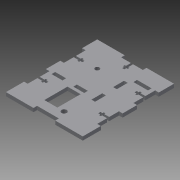
# Autodesk Inventor part: side-right
Saved by Autodesk Inventor 2014 (Build 180170000, 170)
## iProperties
Created: 2014-03-01
Part Number: side-right
Material: 常规
Document SubType Name: Modeling
Designer: Keshuai
Density: 1 g/cm^3
Appearance: 默认
Author: Keshuai
Autodesk Inventor part; units mm, degrees
sketch "slot" plane through (0, 0, 0) normal (0, 0, 1) x (1, 0, 0)
  line L0 (-16.5, 21) -> (-13.5, 21)
  line L1 (-13.5, 9) -> (-16.5, 9)
  line L2 (-11.75, 14.2) -> (-11.75, 11.8)
  line L3 (-18.25, 11.8) -> (-18.25, 14.2)
  line L4 (-18.25, 14.2) -> (-11.75, 11.8) construction
  line L5 (-11.75, 14.2) -> (-18.25, 11.8) construction
  line L6 (-18.25, 14.2) -> (-16.5, 14.2)
  line L7 (-13.5, 14.2) -> (-11.75, 14.2)
  line L8 (-16.5, 9) -> (-16.5, 11.8)
  line L9 (-16.5, 14.2) -> (-16.5, 21)
  line L10 (-13.5, 21) -> (-13.5, 14.2)
  line L11 (-13.5, 11.8) -> (-13.5, 9)
  line L12 (-11.75, 11.8) -> (-13.5, 11.8)
  line L13 (-16.5, 11.8) -> (-18.25, 11.8)
  point P0 (-15, 21)
  point P1 (-15, 13)
  dimension "d33" = 3
  dimension "d34" = 12
  dimension "d35" = 6.5
  dimension "d36" = 2.4
  dimension "d37" = 8
  measures "d33" distance of L11.end L8.start
  measures "d34" distance of L10.start L11.end
  measures "d35" distance of L4.end L5.end
  measures "d36" distance of L5.start L4.end
  measures "d37" distance from line of L0 point (-15, 13)
sketch "草图1" plane through (0, 0, 0) normal (0, 0, 1) x (1, 0, 0)
  line L0 (8, 0) -> (28, 0) projected
  line L1 (28, 0) -> (28, 5) projected
  line L2 (8, 5) -> (28, 5) projected
  line L3 (8, 0) -> (8, 5) projected
  line L4 (33, 0) -> (33, 5) projected
  line L5 (33, 21) -> (-63, 21)
  line L6 (-63, 21) -> (-63, -95)
  line L7 (-63, -95) -> (33, -95)
  line L8 (33, -95) -> (33, 21)
  circle A0 centre (-33, -9) radius 25 construction
  line L9 (0, 0) -> (0, 5) projected
  line L10 (46.5391, -42) -> (-87.8094, -42) construction
  line L11 (-43, -42) -> (-58, -42)
  line L12 (-58, -42) -> (-58, -47)
  line L13 (-58, -47) -> (-43, -47)
  line L14 (-43, -47) -> (-43, -42)
  line L15 (-13, -42) -> (-28, -42)
  line L16 (-28, -42) -> (-28, -47)
  line L17 (-28, -47) -> (-13, -47)
  line L18 (-13, -47) -> (-13, -42)
  line L19 (-9, -106.2504) -> (-9, 32.3829) construction
  line L20 (0, -5) -> (5, -5)
  line L21 (5, -5) -> (5, -20)
  line L22 (5, -20) -> (0, -20)
  line L23 (0, -20) -> (0, -5)
  line L24 (0, -35) -> (5, -35)
  line L25 (5, -35) -> (5, -50)
  line L26 (5, -50) -> (0, -50)
  line L27 (0, -50) -> (0, -35)
  circle A1 centre (-33, -9) radius 3
  dimension "d0" = 16
  dimension "d3" = 50
  dimension "d4" = 30
  dimension "d5" = 33
  dimension "d6" = 30
  dimension "d7" = 33
  dimension "d8" = 53
  dimension "d9" = 15
  dimension "d10" = 5
  dimension "d11" = 15
  dimension "d12" = 5
  dimension "d13" = 5
  dimension "d14" = 15
  dimension "d15" = 54
  dimension "d16" = 5
  dimension "d17" = 15
  dimension "d18" = 5
  dimension "d19" = 15
  dimension "d20" = 5
  dimension "d21" = 15
  dimension "d22" = 6
  constraints: 44 end point, 11 parallel, 6 perpendicular, 5 horizontal, 2 centre point, 2 point on line, 1 coincident, 1 collinear
  measures "d0" distance between parallel lines of L2 L5
  measures "d3" diameter of A0
  measures "d4" distance from line of L5 A0.centre
  measures "d5" distance from line of L9 A0.centre
  measures "d6" distance from line of L6 A0.centre
  measures "d7" distance from line of L10 A0.centre
  measures "d8" distance between parallel lines of L7 L10
  measures "d9" distance of L13.end L12.end
  measures "d10" distance of L12.end L11.end
  measures "d11" distance of L17.end L16.end
  measures "d12" distance of L16.end L15.end
  measures "d13" distance between parallel lines of L6 L12
  measures "d14" distance between parallel lines of L14 L16
  measures "d15" distance between parallel lines of L6 L19
  measures "d16" distance of L21.end L22.end
  measures "d17" distance of L20.end L21.end
  measures "d18" distance of L25.end L26.end
  measures "d19" distance of L24.end L25.end
  measures "d20" distance from line of L20 L9.start
  measures "d21" distance between parallel lines of L24 L22
  measures "d22" diameter of A1
extrude "拉伸1" add sketch "草图1" along normal blind 5
sketch "草图3" plane through (-63, 21, 0) normal (0, 1, 0) x (1, 0, 0)
  line L0 (96, 0) -> (0, 0) projected
  line L1 (0, 0) -> (0, -5) projected
  line L2 (96, -5) -> (0, -5) projected
  line L3 (96, 0) -> (96, -5) projected
  line L4 (74, 10) -> (74, 69)
  line L5 (74, 69) -> (69, 69)
  line L6 (69, 69) -> (69, 10)
  line L7 (69, 10) -> (74, 10)
  circle A0 centre (48, -2.5) radius 1.5
  circle A1 centre (48, 74.5) radius 1.5
  line L8 (0, 72) -> (33, 72)
  line L9 (33, 72) -> (33, 77)
  line L10 (33, 77) -> (63, 77)
  line L11 (63, 77) -> (63, 72)
  line L12 (63, 72) -> (96, 72)
  line L13 (96, 72) -> (96, 0)
  line L14 (96, 0) -> (63, 0)
  line L15 (63, 0) -> (63, -5)
  line L16 (63, -5) -> (33, -5)
  line L17 (33, -5) -> (33, 0)
  line L18 (33, 0) -> (0, 0)
  line L19 (0, 0) -> (0, 72)
  constraints: 32 end point, 8 horizontal, 8 vertical, 2 centre point, 17 other
ref_plane "工作平面1" through (-63, 26, -77) normal (0, 1, 0) x (0, 0, 1)
extrude "拉伸2" add sketch "草图3" along normal up to surface (5 mm away) contours L3 L2 L15 L0 | L17 L2 L1 L0
sketch "草图4" plane through (33, -95, 5) normal (1, 0, 0) x (0, 0, -1)
  line L0 (5, 0) -> (5, 121) projected
  line L1 (5, 121) -> (0, 121) projected
  line L2 (0, 0) -> (0, 121) projected
  line L3 (5, 0) -> (0, 0) projected
  circle A0 centre (41, -2.5) radius 1.5
  circle A1 centre (79.5, 33.5) radius 1.5
  circle A2 centre (79.5, 85) radius 1.5
  circle A3 centre (2.5, 85) radius 1.5
  circle A4 centre (2.5, 35) radius 1.5
  line L4 (77, 70) -> (77, 50)
  line L5 (77, 50) -> (82, 50)
  line L6 (82, 50) -> (82, 20)
  line L7 (82, 20) -> (77, 20)
  line L8 (77, 20) -> (77, 0)
  line L9 (77, 0) -> (56, 0)
  line L10 (56, 0) -> (56, -5)
  line L11 (56, -5) -> (26, -5)
  line L12 (26, -5) -> (26, 0)
  line L13 (26, 0) -> (5, 0)
  line L14 (5, 0) -> (5, 20)
  line L15 (5, 20) -> (0, 20)
  line L16 (0, 20) -> (0, 50)
  line L17 (0, 50) -> (5, 50)
  line L18 (5, 50) -> (5, 70)
  line L19 (5, 70) -> (0, 70)
  line L20 (0, 70) -> (0, 100)
  line L21 (0, 100) -> (5, 100)
  line L22 (5, 100) -> (5, 121)
  line L23 (5, 121) -> (77, 121)
  line L24 (77, 121) -> (77, 100)
  line L25 (77, 100) -> (82, 100)
  line L26 (82, 100) -> (82, 70)
  line L27 (82, 70) -> (77, 70)
  point P0 (5, 95)
  constraints: 48 end point, 12 horizontal, 12 vertical, 5 centre point, 32 other
ref_plane "工作平面2" through (38, -100, -77) normal (1, 0, 0) x (0, 1, 0)
extrude "拉伸3" add sketch "草图4" along normal up to surface (5 mm away) contours L3 L2 L15 L0 | L17 L2 L19 L0 | L21 L2 L1 L0
sketch "草图5" plane through (-63, -95, 0) normal (-1, 0, 0) x (0, 0, 1)
  line L0 (0, 0) -> (0, 121) projected
  line L1 (0, 0) -> (5, 0) projected
  line L2 (5, 0) -> (5, 121) projected
  line L3 (5, 121) -> (0, 121) projected
  circle A0 centre (-36, -2.5) radius 1.5 projected
  circle A1 centre (-74.5, 33.5) radius 1.5 projected
  circle A2 centre (-74.5, 85) radius 1.5 projected
  circle A3 centre (2.5, 85) radius 1.5 projected
  circle A4 centre (2.5, 35) radius 1.5 projected
  line L4 (-72, 20) -> (-77, 20) projected
  line L5 (-72, 0) -> (-72, 20) projected
  line L6 (-51, 0) -> (-72, 0) projected
  line L7 (-51, 0) -> (-51, -5) projected
  line L8 (-51, -5) -> (-21, -5) projected
  line L9 (-21, -5) -> (-21, 0) projected
  line L10 (0, 0) -> (-21, 0) projected
  line L11 (0, 20) -> (0, 0) projected
  line L12 (5, 20) -> (0, 20) projected
  line L13 (5, 50) -> (5, 20) projected
  line L14 (0, 50) -> (5, 50) projected
  line L15 (0, 70) -> (0, 50) projected
  line L16 (5, 70) -> (0, 70) projected
  line L17 (5, 100) -> (5, 70) projected
  line L18 (0, 100) -> (5, 100) projected
  line L19 (0, 121) -> (0, 100) projected
  line L20 (-72, 121) -> (0, 121) projected
  line L21 (-72, 100) -> (-72, 121) projected
  line L22 (-77, 100) -> (-72, 100) projected
  line L23 (-77, 70) -> (-77, 100) projected
  line L24 (-72, 70) -> (-77, 70) projected
  line L25 (-72, 50) -> (-72, 70) projected
  line L26 (-77, 50) -> (-72, 50) projected
  line L27 (-77, 20) -> (-77, 50) projected
  point P0 (0, 95)
ref_plane "工作平面3" through (-68, -100, -77) normal (-1, 0, 0) x (0, 0, 1)
extrude "拉伸4" add sketch "草图5" along normal up to surface (5 mm away) contours L0 L12 L2 L1 | L0 L16 L2 L14 | L0 L3 L2 L18
sketch "草图6" plane through (38, -95, 0) normal (0, -1, 0) x (1, 0, 0)
  line L0 (0, 0) -> (-106, 0) projected
  line L1 (0, 0) -> (0, 5) projected
  line L2 (0, 5) -> (-106, 5) projected
  line L3 (-106, 5) -> (-106, 0) projected
  line L4 (-68, 0) -> (-106, 0) projected
  line L5 (-106, 0) -> (-106, -21) projected
  line L6 (-101, -21) -> (-106, -21) projected
  line L7 (-101, -37.5) -> (-101, -51) projected
  line L8 (-101, -51) -> (-106, -51) projected
  line L9 (-106, -51) -> (-106, -72) projected
  line L10 (-68, -72) -> (-106, -72) projected
  line L11 (-68, -72) -> (-68, -77) projected
  line L12 (-68, -77) -> (-38, -77) projected
  line L13 (-38, -77) -> (-38, -72) projected
  line L14 (-38, -72) -> (0, -72) projected
  line L15 (0, -72) -> (0, -51) projected
  line L16 (-5, -51) -> (0, -51) projected
  line L17 (-5, -34.5) -> (-5, -21) projected
  line L18 (-5, -21) -> (0, -21) projected
  line L19 (0, -21) -> (0, 0) projected
  line L20 (-38, 0) -> (0, 0) projected
  line L21 (-38, 0) -> (-38, 5) projected
  line L22 (-38, 5) -> (-68, 5) projected
  line L23 (-68, 5) -> (-68, 0) projected
  line L24 (-94.2, -37.5) -> (-101, -37.5) projected
  line L25 (-5, -51) -> (-5, -37.5) projected
  line L26 (-5, -37.5) -> (-11.8, -37.5) projected
  line L27 (-11.8, -37.5) -> (-11.8, -39.25) projected
  line L28 (-11.8, -39.25) -> (-14.2, -39.25) projected
  line L29 (-14.2, -39.25) -> (-14.2, -37.5) projected
  line L30 (-14.2, -37.5) -> (-17, -37.5) projected
  line L31 (-17, -37.5) -> (-17, -34.5) projected
  line L32 (-17, -34.5) -> (-14.2, -34.5) projected
  line L33 (-14.2, -34.5) -> (-14.2, -32.75) projected
  line L34 (-14.2, -32.75) -> (-11.8, -32.75) projected
  line L35 (-11.8, -32.75) -> (-11.8, -34.5) projected
  line L36 (-11.8, -34.5) -> (-5, -34.5) projected
  line L37 (-101, -21) -> (-101, -34.5) projected
  line L38 (-101, -34.5) -> (-94.2, -34.5) projected
  line L39 (-94.2, -34.5) -> (-94.2, -32.75) projected
  line L40 (-94.2, -32.75) -> (-91.8, -32.75) projected
  line L41 (-91.8, -32.75) -> (-91.8, -34.5) projected
  line L42 (-91.8, -34.5) -> (-89, -34.5) projected
  line L43 (-89, -34.5) -> (-89, -37.5) projected
  line L44 (-89, -37.5) -> (-91.8, -37.5) projected
  line L45 (-91.8, -37.5) -> (-91.8, -39.25) projected
  line L46 (-91.8, -39.25) -> (-94.2, -39.25) projected
  line L47 (-94.2, -39.25) -> (-94.2, -37.5) projected
ref_plane "工作平面4" through (-68, -100, -77) normal (0, -1, 0) x (1, 0, 0)
extrude "拉伸5" add sketch "草图6" along normal up to surface (5 mm away) contours L0 L21 L2 L1 | L0 L3 L2 L23
sketch "草图7" plane through (0, 0, 5) normal (0, 0, 1) x (1, 0, 0)
  line L0 (0, 21) -> (-30, 21) projected
  line L1 (-63, -25) -> (-63, 5) projected
  line L2 (-63, -75) -> (-63, -45) projected
  line L3 (33, -75) -> (33, -45) projected
  line L4 (33, -25) -> (33, 5) projected
  line L5 (38, -58.5) -> (38, -61.5) projected
  line L6 (38, -8.5) -> (38, -11.5) projected
  line L7 (-16.5, 26) -> (-13.5, 26) projected
  line L8 (-68, -11.5) -> (-68, -8.5) projected
  line L9 (-68, -61.5) -> (-68, -58.5) projected
  line L10 (-16.5, 21) -> (-13.5, 21)
  line L11 (-13.5, 9) -> (-16.5, 9)
  line L12 (-11.75, 14.2) -> (-11.75, 11.8)
  line L13 (-18.25, 11.8) -> (-18.25, 14.2)
  line L14 (-18.25, 14.2) -> (-11.75, 11.8) construction
  line L15 (-11.75, 14.2) -> (-18.25, 11.8) construction
  line L16 (-18.25, 14.2) -> (-16.5, 14.2)
  line L17 (-13.5, 14.2) -> (-11.75, 14.2)
  line L18 (-16.5, 9) -> (-16.5, 11.8)
  line L19 (-16.5, 14.2) -> (-16.5, 21)
  line L20 (-13.5, 21) -> (-13.5, 14.2)
  line L21 (-13.5, 11.8) -> (-13.5, 9)
  line L22 (-11.75, 11.8) -> (-13.5, 11.8)
  line L23 (-16.5, 11.8) -> (-18.25, 11.8)
  line L24 (-63, -61.5) -> (-63, -58.5)
  line L25 (-51, -58.5) -> (-51, -61.5)
  line L26 (-56.2, -56.75) -> (-53.8, -56.75)
  line L27 (-53.8, -63.25) -> (-56.2, -63.25)
  line L28 (-56.2, -63.25) -> (-53.8, -56.75) construction
  line L29 (-56.2, -56.75) -> (-53.8, -63.25) construction
  line L30 (-56.2, -63.25) -> (-56.2, -61.5)
  line L31 (-56.2, -58.5) -> (-56.2, -56.75)
  line L32 (-51, -61.5) -> (-53.8, -61.5)
  line L33 (-56.2, -61.5) -> (-63, -61.5)
  line L34 (-63, -58.5) -> (-56.2, -58.5)
  line L35 (-53.8, -58.5) -> (-51, -58.5)
  line L36 (-53.8, -56.75) -> (-53.8, -58.5)
  line L37 (-53.8, -61.5) -> (-53.8, -63.25)
  line L38 (33, -58.5) -> (33, -61.5)
  line L39 (21, -61.5) -> (21, -58.5)
  line L40 (26.2, -63.25) -> (23.8, -63.25)
  line L41 (23.8, -56.75) -> (26.2, -56.75)
  line L42 (26.2, -56.75) -> (23.8, -63.25) construction
  line L43 (26.2, -63.25) -> (23.8, -56.75) construction
  line L44 (26.2, -56.75) -> (26.2, -58.5)
  line L45 (26.2, -61.5) -> (26.2, -63.25)
  line L46 (21, -58.5) -> (23.8, -58.5)
  line L47 (26.2, -58.5) -> (33, -58.5)
  line L48 (33, -61.5) -> (26.2, -61.5)
  line L49 (23.8, -61.5) -> (21, -61.5)
  line L50 (23.8, -63.25) -> (23.8, -61.5)
  line L51 (23.8, -58.5) -> (23.8, -56.75)
  line L52 (-63, -11.5) -> (-63, -8.5)
  line L53 (-51, -8.5) -> (-51, -11.5)
  line L54 (-56.2, -6.75) -> (-53.8, -6.75)
  line L55 (-53.8, -13.25) -> (-56.2, -13.25)
  line L56 (-56.2, -13.25) -> (-53.8, -6.75) construction
  line L57 (-56.2, -6.75) -> (-53.8, -13.25) construction
  line L58 (-56.2, -13.25) -> (-56.2, -11.5)
  line L59 (-56.2, -8.5) -> (-56.2, -6.75)
  line L60 (-51, -11.5) -> (-53.8, -11.5)
  line L61 (-56.2, -11.5) -> (-63, -11.5)
  line L62 (-63, -8.5) -> (-56.2, -8.5)
  line L63 (-53.8, -8.5) -> (-51, -8.5)
  line L64 (-53.8, -6.75) -> (-53.8, -8.5)
  line L65 (-53.8, -11.5) -> (-53.8, -13.25)
  line L66 (33, -8.5) -> (33, -11.5)
  line L67 (21, -11.5) -> (21, -8.5)
  line L68 (26.2, -13.25) -> (23.8, -13.25)
  line L69 (23.8, -6.75) -> (26.2, -6.75)
  line L70 (26.2, -6.75) -> (23.8, -13.25) construction
  line L71 (26.2, -13.25) -> (23.8, -6.75) construction
  line L72 (26.2, -6.75) -> (26.2, -8.5)
  line L73 (26.2, -11.5) -> (26.2, -13.25)
  line L74 (21, -8.5) -> (23.8, -8.5)
  line L75 (26.2, -8.5) -> (33, -8.5)
  line L76 (33, -11.5) -> (26.2, -11.5)
  line L77 (23.8, -11.5) -> (21, -11.5)
  line L78 (23.8, -13.25) -> (23.8, -11.5)
  line L79 (23.8, -8.5) -> (23.8, -6.75)
  point P0 (0, 0)
  constraints: 4 vertical, 1 horizontal
extrude "拉伸6" cut sketch "草图7" against normal through all
sketch "草图8" plane through (0, 0, 5) normal (0, 0, 1) x (1, 0, 0)
  line L0 (-13, -47) -> (-28, -47) projected
  line L1 (-14, -51) -> (-32, -51)
  line L2 (-32, -51) -> (-32, -83)
  line L3 (-32, -83) -> (-14, -83)
  line L4 (-14, -83) -> (-14, -51)
  line L5 (-57, -47) -> (-60, -47) projected
  point P0 (0, 0)
  dimension "d40" = 18
  dimension "d41" = 32
  dimension "d42" = 28
  dimension "d43" = 4
  constraints: 8 end point, 2 parallel, 1 horizontal, 1 perpendicular
  measures "d40" distance of L3.end L2.end
  measures "d41" distance of L2.end L1.end
  measures "d42" distance from line of L5.end L2
  measures "d43" distance between parallel lines of L1 L0
extrude "拉伸7" cut sketch "草图8" against normal through all
sketch "草图9" plane through (0, 0, 5) normal (0, 0, 1) x (1, 0, 0)
  circle A0 centre (-4.7249, -83) radius 3.6
  point P0 (0, 0)
  dimension "d46" = 7.2
  constraints: 1 centre point
  measures "d46" diameter of A0
extrude "拉伸8" cut sketch "草图9" against normal through all
